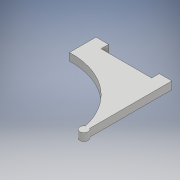
# Autodesk Inventor part: roue_libre
Saved by Autodesk Inventor 2017 (Build 210142000, 142)
## iProperties
Part Number: roue_libre
Material: Générique
Document SubType Name: Modeling
Designer: Thomas
Density: 1 g/cm^3
Appearance: Par défaut
Author: Thomas
Autodesk Inventor part; units mm, degrees
ref_plane "YZ Plane" through (0, 0, 0) normal (1, 0, 0) x (0, 1, 0)
ref_plane "XZ Plane" through (0, 0, 0) normal (0, 1, 0) x (-1, 0, 0)
ref_plane "XY Plane" through (0, 0, 0) normal (0, 0, 1) x (1, 0, 0)
sketch "Esquisse1" plane through (0, 0, 0) normal (0, 0, 1) x (1, 0, 0)
  line L0 (60, 0) -> (60, -65)
  line L1 (0, 0) -> (0, -6)
  arc A0 (56.6718, -65) -> (60, -65) centre (58.3359, -67.8823) ccw
  line L2 (0, 0) -> (10, 0)
  line L3 (10, 0) -> (10, -6)
  line L4 (10, -6) -> (50, -6)
  line L5 (50, -6) -> (50, 0)
  line L6 (0, 0) -> (10, 0)
  line L7 (50, 0) -> (60, 0)
  line L8 (0, -6) -> (0, -21)
  arc A1 (56.6718, -65) -> (0, -21) centre (1.6431, -77.3802) ccw
  dimension "d0" = 60
  dimension "d1" = 65
  dimension "d2" = 6
  dimension "d5" = 10
  dimension "d6" = 10
  dimension "d8" = 15
  constraints: 18 end point, 4 perpendicular, 4 point on circle, 3 vertical, 2 centre point, 2 horizontal
  measures "d0" distance of L1.start L0.start
  measures "d1" distance of L0.start L0.end
  measures "d2" distance of L1.start L1.end
  measures "d5" distance of L1.start L2.end
  measures "d6" distance between parallel lines of L0 L5
  measures "d8" distance of L1.end L8.end
extrude "Extrusion1" add sketch "Esquisse1" along normal blind 6
